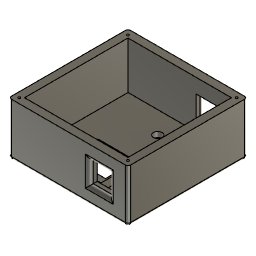
BuzzerClientTop (Autodesk Fusion 360 design; units mm, degrees)
Autodesk Fusion 360 part; units mm, degrees
note: some values were not read from the file. Set by a fixed rule: which sketch regions a step uses.
sketch "Sketch13" plane through (0, 0, 0) normal (0, 0, 1) x (1, 0, 0)
  line L0 (45.45, 45.45) -> (-45.45, 45.45)
  line L1 (-45.45, 45.45) -> (-45.45, -45.45)
  line L2 (-45.45, -45.45) -> (45.45, -45.45)
  line L3 (45.45, -45.45) -> (45.45, 45.45)
  line L4 (45.45, 45.45) -> (-45.45, -45.45) construction
  line L5 (-45.45, 45.45) -> (45.45, -45.45) construction
  dimension "d87" = 90.9
  dimension "d88" = 90.9
  constraint horizontal L0
  constraint perpendicular L0 L1
  constraint parallel L0 L2
  constraint parallel L1 L3
  constraint coincident L4 origin
  constraint coincident L5 origin
  measures "d87" distance of L1.end L2.end
  measures "d88" distance of L0.end L1.end
extrude "Extrude12" add sketch "Sketch13" along normal blind 40
sketch "Sketch14" plane through (0, 0, 40) normal (0, 0, 1) x (-1, 0, 0)
  line L0 (-45.45, 45.45) -> (-45.45, -45.45)
  line L1 (-45.45, -45.45) -> (45.45, -45.45)
  line L2 (45.45, -45.45) -> (45.45, 45.45)
  line L3 (45.45, 45.45) -> (-45.45, 45.45)
  line L4 (-39.45, -39.45) -> (39.45, -39.45)
  line L5 (39.45, -39.45) -> (39.45, 39.45)
  line L6 (39.45, 39.45) -> (-39.45, 39.45)
  line L7 (-39.45, 39.45) -> (-39.45, -39.45)
  line L8 (-39.45, -39.45) -> (39.45, 39.45) construction
  line L9 (39.45, -39.45) -> (-39.45, 39.45) construction
  dimension "d91" = 78.9
  dimension "d92" = 78.9
  constraint horizontal L4
  constraint perpendicular L4 L5
  constraint parallel L4 L6
  constraint parallel L5 L7
  constraint coincident L8 origin
  constraint coincident L9 origin
  measures "d91" distance of L5.end L6.end
  measures "d92" distance of L4.end L5.end
extrude "Extrude13" cut sketch "Sketch14" against normal blind 36 contours L4 L5 L6 L7
sketch "Sketch15" plane through (0, 0, 40) normal (0, 0, 1) x (-1, 0, 0)
  line L0 (39.45, -39.45) -> (-39.45, -39.45)
  line L1 (-39.45, -39.45) -> (-39.45, 39.45)
  line L2 (-39.45, 39.45) -> (39.45, 39.45)
  line L3 (39.45, 39.45) -> (39.45, -39.45)
  line L4 (-45.45, 45.45) -> (-45.45, -45.45)
  line L5 (-45.45, -45.45) -> (45.45, -45.45)
  line L6 (45.45, -45.45) -> (45.45, 45.45)
  line L7 (45.45, 45.45) -> (-45.45, 45.45)
  line L8 (45.45, -45.45) -> (41.45, -45.45)
  line L9 (45.45, -41.45) -> (45.45, -45.45)
  circle A0 centre (41.45, -41.45) radius 0.85
  line L10 (-45.45, -45.45) -> (-41.45, -45.45)
  line L11 (-45.45, -41.45) -> (-45.45, -45.45)
  circle A1 centre (-41.45, -41.45) radius 0.85
  line L12 (45.45, 45.45) -> (41.45, 45.45)
  line L13 (41.45, 45.45) -> (41.45, 42.3)
  line L14 (45.45, 41.45) -> (45.45, 45.45)
  circle A2 centre (41.45, 41.45) radius 0.85
  line L15 (-45.45, 45.45) -> (-41.45, 45.45)
  line L16 (-45.45, 41.45) -> (-45.45, 45.45)
  circle A3 centre (-41.45, 41.45) radius 0.85
  line L17 (-41.45, 45.45) -> (-41.45, 42.3)
  line L18 (-42.3, 41.45) -> (-45.45, 41.45)
  line L19 (42.3, 41.45) -> (45.45, 41.45)
  line L20 (41.45, -45.45) -> (41.45, -42.3)
  line L21 (42.3, -41.45) -> (45.45, -41.45)
  line L22 (-41.45, -45.45) -> (-41.45, -42.3)
  line L23 (-42.3, -41.45) -> (-45.45, -41.45)
  dimension "d95" = 4
  dimension "d96" = 4
  dimension "d97" = 1.7
  dimension "d98" = 4
  dimension "d99" = 4
  dimension "d100" = 1.7
  dimension "d101" = 4
  dimension "d102" = 4
  dimension "d103" = 1.7
  dimension "d104" = 4
  dimension "d105" = 4
  dimension "d106" = 1.7
  constraint horizontal L8
  constraint vertical L9
  constraint coincident L5.end L6.start
  constraint horizontal L10
  constraint vertical L11
  constraint coincident L4.end L5.start
  constraint horizontal L12
  constraint vertical L13
  constraint vertical L14
  constraint coincident L6.end L7.start
  constraint horizontal L15
  constraint vertical L16
  constraint coincident L4.start L7.end
  constraint coincident A3 L17.end
  constraint vertical L17
  constraint coincident A3 L18.start
  constraint horizontal L18
  constraint coincident A2 L19.start
  constraint horizontal L19
  constraint coincident A2 L13.end
  constraint coincident A0 L20.end
  constraint vertical L20
  constraint coincident A0 L21.start
  constraint horizontal L21
  constraint coincident A1 L22.end
  constraint vertical L22
  constraint coincident A1 L23.start
  constraint horizontal L23
  measures "d95" distance of L5.end L8.end
  measures "d96" distance of L5.end L9.start
  measures "d97" diameter of A0
  measures "d98" distance of L4.end L10.end
  measures "d99" distance of L4.end L11.start
  measures "d100" diameter of A1
  measures "d101" distance of L6.end L12.end
  measures "d102" distance of L6.end L14.start
  measures "d103" diameter of A2
  measures "d104" distance of L4.start L15.end
  measures "d105" distance of L4.start L16.start
  measures "d106" diameter of A3
extrude "Extrude14" cut sketch "Sketch15" against normal blind 20 contours A3 | A1 | A2 | A0
sketch "Sketch16" plane through (0, 0, 0) normal (0, 0, 1) x (1, 0, 0)
  circle A0 centre (0, 22.6858) radius 3.35
  line L0 (0, 45.4608) -> (0, 26.0358)
  line L1 (0, 19.3358) -> (0, -8.7142)
  line L2 (16, -8.7142) -> (-14, -8.7142)
  line L3 (-14, -8.7142) -> (-14, -36.7142)
  line L4 (-14, -36.7142) -> (16, -36.7142)
  line L5 (16, -36.7142) -> (16, -8.7142)
  point P0 (0, -22.7142)
  dimension "d109" = 22.775
  dimension "d110" = 6.7
  dimension "d138" = 45.4
  dimension "d139" = 30
  dimension "d140" = 28
  constraint coincident A0 L0.end
  constraint vertical L0
  constraint vertical L1
  constraint coincident A0 L1.start
  constraint horizontal L2
  constraint perpendicular L2 L3
  constraint parallel L2 L4
  constraint parallel L3 L5
  constraint coincident L2 L1.end
  measures "d109" distance of L0.start A0.centre
  measures "d110" diameter of A0
  measures "d138" distance of A0.centre P0
  measures "d139" distance of L3.end L4.end
  measures "d140" distance of L2.end L3.end
extrude "Extrude15" cut sketch "Sketch16" along normal blind 4 contours A0
sketch "Sketch17" plane through (0, -39.45, 0) normal (0, 1, 0) x (-1, 0, 0)
  line L0 (39.45, 40) -> (-39.45, 40)
  line L1 (-39.45, 40) -> (-39.45, 4)
  line L2 (39.45, 4) -> (39.45, 40)
  line L3 (-39.45, 40) -> (-32.355, 40)
  line L4 (-32.355, 40) -> (-32.355, 29)
  line L5 (-32.355, 29) -> (-39.45, 29)
  line L6 (-39.45, 29) -> (-39.45, 40)
  line L7 (-32.355, 29) -> (-31.155, 29)
  line L8 (-31.155, 29) -> (-15.955, 29)
  line L9 (-15.955, 29) -> (-15.955, 14.4)
  line L10 (-31.155, 14.4) -> (-31.155, 29)
  line L11 (-31.155, 14.4) -> (-31.155, 12.4)
  line L12 (-31.155, 12.4) -> (-15.955, 12.4)
  line L13 (-15.955, 12.4) -> (-15.955, 14.4)
  line L14 (-39.45, 4) -> (39.45, 4)
  dimension "d113" = 7.095
  dimension "d114" = 11
  dimension "d115" = 1.2
  dimension "d116" = 15.2
  dimension "d117" = 14.6
  dimension "d248" = 2
  constraint horizontal L3
  constraint vertical L4
  constraint horizontal L5
  constraint vertical L6
  constraint coincident L0.end L1.start
  constraint perpendicular L4 L7
  constraint horizontal L8
  constraint vertical L9
  constraint vertical L10
  constraint vertical L11
  constraint horizontal L12
  constraint vertical L13
  measures "d113" distance of L0.end L3.end
  measures "d114" distance of L0.end L5.end
  measures "d115" distance of L4.end L7.end
  measures "d116" distance of L7.end L8.end
  measures "d117" distance of L7.end L10.start
  measures "d248" distance of L9.end L12.end
extrude "Extrude16" cut sketch "Sketch17" against normal blind 10 contours L8 L9 L10 L11 L12 L13
sketch "Sketch18" plane through (0, 39.45, 0) normal (0, -1, 0) x (1, 0, 0)
  line L0 (39.45, 40) -> (-39.45, 40)
  line L1 (-39.45, 40) -> (-39.45, 4)
  line L2 (39.45, 4) -> (39.45, 40)
  line L3 (39.45, 40) -> (28.92, 40)
  line L4 (28.92, 40) -> (28.92, 29)
  line L5 (28.92, 29) -> (39.45, 29)
  line L6 (39.45, 29) -> (39.45, 40)
  line L7 (28.92, 29) -> (27.72, 29)
  line L8 (27.72, 29) -> (12.52, 29)
  line L9 (12.52, 29) -> (12.52, 14.4)
  line L10 (27.72, 14.4) -> (27.72, 29)
  line L11 (27.72, 14.4) -> (27.72, 12.4)
  line L12 (27.72, 12.4) -> (12.52, 12.4)
  line L13 (12.52, 12.4) -> (12.52, 14.4)
  line L14 (-39.45, 4) -> (39.45, 4)
  dimension "d120" = 10.53
  dimension "d121" = 11
  dimension "d122" = 1.2
  dimension "d123" = 15.2
  dimension "d124" = 14.6
  dimension "d249" = 2
  constraint horizontal L3
  constraint vertical L4
  constraint horizontal L5
  constraint vertical L6
  constraint coincident L0.start L2.end
  constraint perpendicular L4 L7
  constraint horizontal L8
  constraint vertical L9
  constraint vertical L10
  constraint vertical L11
  constraint horizontal L12
  constraint vertical L13
  measures "d120" distance of L0.start L3.end
  measures "d121" distance of L0.start L5.end
  measures "d122" distance of L4.end L7.end
  measures "d123" distance of L7.end L8.end
  measures "d124" distance of L7.end L10.start
  measures "d249" distance of L9.end L12.end
extrude "Extrude17" cut sketch "Sketch18" against normal blind 10 contours L8 L9 L10 L11 L12 L13
fillet "Fillet1" radius 2 8 edges at (45.45, -45.45, 20) (45.45, 0, 0) (0, -45.45, 0) (-45.45, -45.45, 20) (45.45, 45.45, 20) (-45.45, 45.45, 20) (-45.45, 0, 0) (0, 45.45, 0)
extrude "Extrude19" add sketch "Sketch16" along normal blind 10 contours L2 L3 L4 L5
sketch "Sketch20" plane through (0, 0, 10) normal (0, 0, 1) x (-1, 0, 0)
  line L0 (-16, 36.7142) -> (-16, 8.7142)
  line L1 (-16, 8.7142) -> (14, 8.7142)
  line L2 (14, 8.7142) -> (14, 36.7142)
  line L3 (14, 36.7142) -> (-16, 36.7142)
  line L4 (-14.8, 32) -> (12.5, 32)
  line L5 (12.5, 32) -> (12.5, 12.7)
  line L6 (12.5, 12.7) -> (-14.8, 12.7)
  line L7 (-14.8, 12.7) -> (-14.8, 32)
  line L8 (-14.8, 32) -> (12.5, 12.7) construction
  line L9 (12.5, 32) -> (-14.8, 12.7) construction
  point P0 (-1.15, 22.35)
  dimension "d143" = 27.3
  dimension "d144" = 19.3
  constraint horizontal L4
  constraint perpendicular L4 L5
  constraint parallel L4 L6
  constraint parallel L5 L7
  constraint coincident L8 P0
  constraint coincident L9 P0
  measures "d143" distance of L5.end L6.end
  measures "d144" distance of L4.end L5.end
extrude "Extrude20" cut sketch "Sketch20" against normal blind 10 contours L4 L5 L6 L7
sketch "Sketch21" plane through (0, 0, 10) normal (0, 0, 1) x (-1, 0, 0)
  line L0 (12.5, 32) -> (12.5, 12.7)
  line L1 (12.5, 12.7) -> (-14.8, 12.7)
  line L2 (-14.8, 12.7) -> (-14.8, 32)
  line L3 (-14.8, 32) -> (12.5, 32)
  line L4 (-16, 36.7142) -> (-16, 8.7142)
  line L5 (-16, 8.7142) -> (14, 8.7142)
  line L6 (14, 8.7142) -> (14, 36.7142)
  line L7 (14, 36.7142) -> (-16, 36.7142)
  line L8 (12.5, 12.7) -> (11, 12.7)
  line L9 (11, 12.7) -> (11, 11.65)
  line L10 (11.75, 11.2) -> (12.5, 11.2)
  line L11 (12.5, 11.2) -> (12.5, 12.7)
  circle A0 centre (11, 10.8) radius 0.85
  circle A1 centre (-11.7, 10.8) radius 0.85
  line L12 (12.5, 32) -> (11, 32)
  line L13 (11, 32) -> (11, 32.65)
  line L14 (11.85, 33.5) -> (12.5, 33.5)
  line L15 (12.5, 33.5) -> (12.5, 32)
  circle A2 centre (11, 33.5) radius 0.85
  circle A3 centre (-11.7, 33.5) radius 0.85
  line L16 (11, 10.8) -> (-11.7, 10.8)
  dimension "d147" = 1.5
  dimension "d148" = 1.5
  dimension "d149" = 1.7
  dimension "d155" = 1.7
  dimension "d156" = 1.5
  dimension "d157" = 1.5
  dimension "d158" = 1.7
  dimension "d159" = 22.7
  dimension "d160" = 1.7
  dimension "d167" = 22.7
  dimension "d193" = 22.7
  constraint horizontal L8
  constraint vertical L9
  constraint horizontal L10
  constraint vertical L11
  constraint coincident L0.end L1.start
  constraint coincident A0 L9.end
  constraint coincident A0 L10.start
  constraint horizontal L12
  constraint vertical L13
  constraint horizontal L14
  constraint vertical L15
  constraint coincident L0.start L3.end
  constraint coincident A2 L13.end
  constraint coincident A2 L14.start
  constraint coincident A0.centre L16.start
  constraint horizontal L16
  constraint coincident A1.centre L16.end
  measures "d147" distance of L0.end L8.end
  measures "d148" distance of L0.end L10.end
  measures "d149" diameter of A0
  measures "d155" diameter of A1
  measures "d156" distance of L0.start L12.end
  measures "d157" distance of L0.start L14.end
  measures "d158" diameter of A2
  measures "d159" distance of A2.centre A3.centre
  measures "d160" diameter of A3
  measures "d167" distance of A0.centre A1.centre
  measures "d193" distance of A0.centre A2.centre
sketch "Sketch23" plane through (0, 0, 10) normal (0, 0, 1) x (-1, 0, 0)
  line L0 (12.5, 32) -> (12.5, 12.7)
  line L1 (12.5, 12.7) -> (-14.8, 12.7)
  line L2 (-14.8, 12.7) -> (-14.8, 32)
  line L3 (-16, 36.7142) -> (-16, 8.7142)
  line L4 (-16, 8.7142) -> (14, 8.7142)
  line L5 (14, 8.7142) -> (14, 36.7142)
  line L6 (14, 36.7142) -> (-16, 36.7142)
  line L7 (11, 33.5) -> (6.5, 33.5)
  line L8 (-11.7, 33.5) -> (-7.2, 33.512)
  line L9 (6.5, 33.5) -> (6.5, 36.7142)
  line L10 (-7.2, 33.512) -> (-7.2, 32.9957)
  line L11 (6.5, 36.7142) -> (-7.2, 36.7142)
  line L12 (-7.2, 36.7142) -> (-7.2, 32.9957)
  line L13 (-7.2, 32.9957) -> (6.5, 32.9957)
  line L14 (6.5, 32.9957) -> (6.5, 36.7142)
  line L15 (6.5, 32.9957) -> (-7.2, 32.9957)
  line L16 (6.5, 32) -> (6.5, 33)
  dimension "d170" = 4.5
  dimension "d171" = 4.5
  dimension "d206" = 1
  constraint horizontal L7
  constraint coincident L6 L9.end
  constraint perpendicular L6 L9
  constraint horizontal L11
  constraint vertical L12
  constraint horizontal L13
  constraint vertical L14
  constraint horizontal L15
  constraint vertical L16
  measures "d170" distance of L7.start L7.end
  measures "d171" distance of L8.start L8.end
  measures "d206" distance of L16.start L16.end
extrude "Extrude29" cut sketch "Sketch23" against normal blind 4 contours L6 L9 L10 L11 L12 L13 L14 L15 L16
extrude "Extrude24" cut sketch "Sketch23" against normal blind 5 contours L6 L9 L10 L11 L12 L13 L14 L15 L16
fillet "Fillet3" radius 2 4 edges at (1.15, -12.7, 0) (14.8, -22.35, 0) (1.15, -32, 0) (-12.5, -22.35, 0)
fillet "Fillet8" radius 3 4 edges at (12.52, 45.45, 20.7) (20.12, 45.45, 29) (27.72, 45.45, 20.7) (20.12, 45.45, 12.4)
fillet "Fillet9" radius 3 4 edges at (31.155, -45.45, 20.7) (23.555, -45.45, 29) (15.955, -45.45, 20.7) (23.555, -45.45, 12.4)
